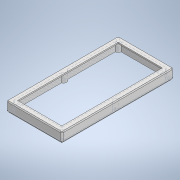
# Autodesk Inventor part: Cover
Saved by Autodesk Inventor 2021 (Build 250183000, 183)
## iProperties
Created: 2020-07-20
Part Number: Cover
Material: Generic
Document SubType Name: Modeling
Designer: ameli
Density: 1 g/cm^3
Appearance: Default
Author: ameli
Autodesk Inventor part; units mm, degrees
ref_plane "YZ Plane" through (0, 0, 0) normal (1, 0, 0) x (0, 1, 0)
ref_plane "XZ Plane" through (0, 0, 0) normal (0, 1, 0) x (-1, 0, 0)
ref_plane "XY Plane" through (0, 0, 0) normal (0, 0, 1) x (1, 0, 0)
sketch "Sketch1" plane through (0, 0, 0) normal (0, 1, 0) x (-1, 0, 0)
  line L0 (66.5, 134) -> (-66.5, 134)
  line L1 (-66.5, 134) -> (-66.5, -134)
  line L2 (-66.5, -134) -> (66.5, -134)
  line L3 (66.5, -134) -> (66.5, 134)
  point P0 (0, 0)
  dimension "d0" = 133
  dimension "d1" = 268
  dimension "d2" = 66.5
  dimension "d3" = 134
  constraints: 8 end point, 2 parallel, 1 horizontal, 1 perpendicular
  measures "d0" distance of L0.start L0.end
  measures "d1" distance of L2.end L0.start
  measures "d2" distance from line of point (0, 0) L3
  measures "d3" distance from line of point (0, 0) L0
extrude "Extrusion1" add sketch "Sketch1" along normal blind 20.3
shell "Shell1" thickness 3 removed faces 1 at (-22.1667, 0, -44.6667)
sketch "Sketch2" plane through (0, 20.3, 0) normal (0, 1, 0) x (1, 0, 0)
  line L0 (-53, 120.5) -> (53, 120.5)
  line L1 (53, 120.5) -> (53, -120.5)
  line L2 (53, -120.5) -> (-53, -120.5)
  line L3 (-53, -120.5) -> (-53, 120.5)
  line L4 (-66.5, 134) -> (-66.5, -134) projected
  line L5 (-66.5, -134) -> (66.5, -134) projected
  line L6 (66.5, -134) -> (66.5, 134) projected
  line L7 (66.5, 134) -> (-66.5, 134) projected
  point P0 (0, 0)
  dimension "d7" = 13.5
  dimension "d8" = 13.5
  dimension "d9" = 13.5
  dimension "d10" = 13.5
  constraints: 8 end point, 2 parallel, 1 horizontal, 1 perpendicular
  measures "d7" distance between parallel lines of L3 L4
  measures "d8" distance between parallel lines of L5 L2
  measures "d9" distance between parallel lines of L6 L1
  measures "d10" distance between parallel lines of L7 L0
extrude "Extrusion2" cut sketch "Sketch2" against normal through all contours L0 L1 L2 L3
sketch "Sketch3" plane through (-63.5, 17.3, 131) normal (0, -1, 0) x (1, 0, 0)
  arc A0 (117, 0) -> (127, -10) centre (127, 0) ccw
  line L0 (127, 0) -> (127, -262) projected
  line L1 (0, 0) -> (127, 0) projected
  line L2 (127, -262) -> (0, -262) projected
  arc A1 (127, -252) -> (117, -262) centre (127, -262) ccw
  line L3 (0, -262) -> (0, 0) projected
  arc A2 (0, -10) -> (10, 0) centre (0, 0) ccw
  arc A3 (10, -262) -> (0, -252) centre (0, -262) ccw
  arc A4 (127, -123.5) -> (127, -138.5) centre (127, -131) ccw
  arc A5 (0, -138.5) -> (0, -123.5) centre (0, -131) ccw
  line L4 (127, 0) -> (124.6095, 0)
  line L5 (127, 0) -> (124.5, 0)
  line L6 (124.5, 0) -> (124.5, -262)
  line L7 (124.5, -262) -> (127, -262)
  line L8 (127, -262) -> (127, 0)
  line L9 (0, 0) -> (2.5, 0)
  line L10 (2.5, 0) -> (2.5, -262)
  line L11 (2.5, -262) -> (0, -262)
  line L12 (0, -262) -> (0, 0)
  line L13 (0, -262) -> (0, 0) projected
  line L14 (0, -262) -> (127, -262)
  line L15 (127, -262) -> (127, -259.5)
  line L16 (127, -259.5) -> (0, -259.5)
  line L17 (0, -259.5) -> (0, -262)
  line L18 (0, 0) -> (127, 0)
  line L19 (127, 0) -> (127, -2.5)
  line L20 (127, -2.5) -> (0, -2.5)
  line L21 (0, -2.5) -> (0, 0)
  point P0 (63.5, -131)
  point P1 (9.6825, -259.5)
  point P2 (2.5, -252.3175)
  point P3 (2.5, -138.0711)
  point P4 (2.5, -123.9289)
  point P5 (2.5, -9.6825)
  point P6 (9.6825, -2.5)
  point P7 (117.3175, -2.5)
  point P8 (124.5, -9.6825)
  point P9 (124.5, -123.9289)
  point P10 (124.5, -138.0711)
  point P11 (124.5, -252.3175)
  point P12 (117.3175, -259.5)
  dimension "d13" = 20
  dimension "d14" = 0
  dimension "d15" = 0
  dimension "d16" = 20
  dimension "d17" = 20
  dimension "d18" = 20
  dimension "d19" = 15
  dimension "d20" = 15
  dimension "d21" = 0
  dimension "d22" = 0
  dimension "d24" = 0
  dimension "d25" = 0
  dimension "d28" = 2.5
  dimension "d29" = 0
  dimension "d30" = 0
  dimension "d31" = 0
  dimension "d32" = 2.5
  dimension "d33" = 0
  dimension "d34" = 2.5
  dimension "d35" = 0
  dimension "d36" = 2.5
  dimension "d37" = 0
  constraints: 34 end point, 12 point on circle, 12 point on line, 8 parallel, 6 centre point, 5 horizontal, 4 perpendicular, 3 coincident
  measures "d13" diameter of A0
  measures "d14" distance from line of L0 A0.centre
  measures "d15" distance from line of L1 A0.centre
  measures "d16" diameter of A1
  measures "d17" diameter of A2
  measures "d18" diameter of A3
  measures "d19" diameter of A4
  measures "d20" diameter of A5
  measures "d21" distance from line of L0 A4.centre
  measures "d22" distance from line of L3 A5.centre
  measures "d24" vertical distance of point (63.5, -131) A4.centre
  measures "d25" vertical distance of point (63.5, -131) A5.centre
  measures "d28" distance of L6.end L7.end
  measures "d29" distance between parallel lines of L0 L8
  measures "d30" distance between parallel lines of L2 L7
  measures "d31" distance between parallel lines of L1 L5
  measures "d32" distance of L10.end L11.end
  measures "d33" distance between parallel lines of L2 L11
  measures "d34" distance of L14.end L15.end
  measures "d35" distance between parallel lines of L0 L15
  measures "d36" distance of L18.end L19.end
  measures "d37" distance between parallel lines of L0 L19
extrude "Extrusion3" add sketch "Sketch3" along normal blind 21.3 contours L1 L6 L20 A0 | A0 L20 A2 L1 | L20 L6 A0 | A2 L20 L10 L1 | L1 L0 L20 L6 | L6 L20 L0 A0 | A0 L0 A4 L6 | A2 L10 L20 | L10 L20 L3 L1 | L6 A4 | A4 L0 L6 | L10 A5 L3 A2 | A2 L3 L20 L10 | A4 L0 A1 L6 | L10 A5 L3 | A5 L10 | L6 L16 A1 | A1 L0 L16 L6 | L10 A3 L3 A5 | L16 L6 L2 A1 | A1 L2 A3 L16 | L16 L0 L2 L6 | L10 L16 L3 A3 | A3 L16 L10 | A3 L2 L10 L16 | L10 L2 L3 L16
fillet "Fillet2" radius 4 4 edges at (-66.5, 10.15, -134) (-66.5, 10.15, 134) (66.5, 10.15, 134) (66.5, 10.15, -134)
fillet "Fillet3" radius 1 4 edges at (53, 18.8, 120.5) (53, 18.8, -120.5) (-53, 18.8, -120.5) (-53, 18.8, 120.5)
chamfer "Chamfer1" distance 2 angle 45 8 edges at (0, 20.3, 134) (65.3284, 20.3, 132.8284) (66.5, 20.3, 0) (65.3284, 20.3, -132.8284) (0, 20.3, -134) (-65.3284, 20.3, -132.8284) (-66.5, 20.3, 0) (-65.3284, 20.3, 132.8284)
sketch "Sketch4" plane through (-63.5, -4, 131) normal (0, -1, 0) x (1, 0, 0)
  circle A0 centre (123.75, -258.75) radius 1.75 projected
  circle A1 centre (3.25, -258.75) radius 1.75 projected
  circle A2 centre (3.25, -3.25) radius 1.75 projected
  circle A3 centre (123.75, -3.25) radius 1.75 projected
  circle A4 centre (123.75, -131) radius 1.75 projected
  circle A5 centre (3.25, -131) radius 1.75 projected
  point P0 (63.5, -131)
  constraints: 6 coincident
hole "Hole1" at (-60.25, -4, 127.75) at (60.25, -4, 127.75) at (60.25, -4, 0) at (60.25, -4, -127.75) at (-60.25, -4, -127.75) at (-60.25, -4, 0) direction (0, 1, 0) diameter 2.6 depth 6 tip angle 118
body "Solid1"
